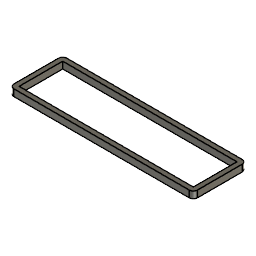
Front clock pice (Autodesk Fusion 360 design; units mm, degrees)
part number: 2026-01-20-20-36-04-765
Autodesk Fusion 360 part; units mm, degrees
sketch "Sketch1" plane through (0, 0, 0) normal (0, 0, 1) x (1, 0, 0)
  line L0 (0, 0) -> (135, 0)
  line L1 (135, 0) -> (135, 39)
  line L2 (135, 39) -> (0, 39)
  line L3 (0, 39) -> (0, 0)
  line L4 (3.5, 35.5) -> (131.5, 35.5)
  line L5 (131.5, 35.5) -> (131.5, 3.5)
  line L6 (131.5, 3.5) -> (3.5, 3.5)
  line L7 (3.5, 3.5) -> (3.5, 35.5)
  dimension "d1" = 135
  dimension "d2" = 128
  dimension "d3" = 32
  dimension "d4" = 39
  dimension "d5" = 3.5
  dimension "d6" = 3.5
  constraint horizontal L0
  constraint vertical L1
  constraint horizontal L2
  constraint vertical L3
  constraint coincident L0.start L3.end
  constraint horizontal L4
  constraint vertical L5
  constraint horizontal L6
  constraint vertical L7
  measures "d1" distance of L0.start L0.end
  measures "d2" distance of L5.end L6.end
  measures "d3" distance of L4.start L6.end
  measures "d4" distance of L0.start L2.end
  measures "d5" distance of L2 L4
  measures "d6" distance of L3 L7
extrude "Extrude1" add sketch "Sketch1" along normal blind 5
fillet "Fillet1" radius 3 4 edges at (0, 0, 2.5) (135, 0, 2.5) (135, 39, 2.5) (0, 39, 2.5)
